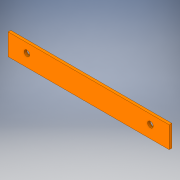
# Autodesk Inventor part: 2018 Cube Backstop Mount
Saved by Autodesk Inventor 2018 (Build 220112000, 112)
## iProperties
Created: 2018-01-23
Part Number: 2018 Cube Backstop Mount
Material: Generic
Document SubType Name: Modeling
Designer: Apple
Density: 1 g/cm^3
Appearance: Default
Author: Apple
Autodesk Inventor part; units mm, degrees
ref_plane "YZ Plane" through (0, 0, 0) normal (1, 0, 0) x (0, 1, 0)
ref_plane "XZ Plane" through (0, 0, 0) normal (0, 1, 0) x (-1, 0, 0)
ref_plane "XY Plane" through (0, 0, 0) normal (0, 0, 1) x (1, 0, 0)
sketch "Sketch1" plane through (0, 0, 0) normal (0, 0, 1) x (1, 0, 0)
  line L0 (-92.075, -25.4) -> (92.075, -25.4)
  line L1 (95.25, -3.9116) -> (-95.25, -3.9116)
  line L2 (-95.25, -3.9116) -> (-95.25, -29.3116)
  line L3 (-95.25, -29.3116) -> (95.25, -29.3116)
  line L4 (95.25, -29.3116) -> (95.25, -3.9116)
  point P0 (0, 0)
  dimension "d5" = 25.4
  constraints: 10 end point, 2 parallel, 1 horizontal, 1 perpendicular, 2 other
  measures "d5" distance of L1.end L2.end
extrude "Extrusion1" add sketch "Sketch1" along normal blind 3.175
sketch "Sketch2" plane through (0, 0, 3.175) normal (0, 0, 1) x (1, 0, 0)
  arc A0 (82.55, -18.034) -> (82.55, -11.2776) centre (82.55, -14.6558) ccw
  arc A1 (-82.55, -11.2776) -> (-82.55, -18.034) centre (-82.55, -14.6558) ccw
  line L0 (-63.5, -11.2776) -> (-82.55, -11.2776)
  arc A2 (-63.5, -18.034) -> (-63.5, -11.2776) centre (-63.5, -14.6558) ccw
  line L1 (-82.55, -18.034) -> (-63.5, -18.034)
  line L2 (63.5, -18.034) -> (82.55, -18.034)
  arc A3 (63.5, -11.2776) -> (63.5, -18.034) centre (63.5, -14.6558) ccw
  line L3 (82.55, -11.2776) -> (63.5, -11.2776)
  circle A4 centre (73.025, -14.6558) radius 3.3782
  circle A5 centre (-73.025, -14.6558) radius 3.3782
  line L4 (95.25, -3.9116) -> (-95.25, -3.9116) projected
  point P0 (0, 0)
  dimension "d4" = 10.7442
  constraints: 8 end point, 8 point on circle, 6 centre point, 1 horizontal alignment
  measures "d4" distance from line of L4 A5.centre
extrude "Extrusion2" cut sketch "Sketch2" against normal through all contours A4 | A5
body "Solid1"
